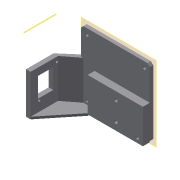
# Autodesk Inventor part: cellSTORM_inverted_Laser_left
Saved by Autodesk Inventor 2019.4 (Build 234330000, 330)
## iProperties
Created: 2020-11-05
Part Number: cellSTORM_inverted_Laser_left
Material: Generic
Document SubType Name: Modeling
Designer: diederichbenedict
Density: 1 g/cm^3
Appearance: Default
Author: diederichbenedict
Autodesk Inventor part; units mm, degrees
ref_plane "Work Plane1" through (0, 0, 0) normal (0, 0, 1) x (1, 0, 0)
sketch "Sketch1" plane through (0, 0, 0) normal (0, 0, 1) x (1, 0, 0)
  circle A0 centre (0, 25) radius 1.95 construction
  circle A1 centre (-25, 0) radius 1.95 construction
  circle A2 centre (-25, -25) radius 1.95 construction
  circle A3 centre (25, 25) radius 1.95 construction
  circle A4 centre (25, -25) radius 1.95 construction
  circle A5 centre (-25, 25) radius 1.95 construction
  circle A6 centre (25, 0) radius 1.95 construction
  circle A7 centre (0, -25) radius 1.95 construction
  line L0 (-28, 30) -> (-30, 28) projected
  line L1 (-30, 28) -> (-30, -28) projected
  line L2 (-30, -28) -> (-28, -30) projected
  line L3 (-28, -30) -> (28, -30) projected
  line L4 (28, -30) -> (30, -28) projected
  line L5 (30, -28) -> (30, 28) projected
  line L6 (30, 28) -> (28, 30) projected
  line L7 (28, 30) -> (-28, 30) projected
  circle A8 centre (25, 25) radius 1.45
  circle A9 centre (25, -25) radius 1.45
  circle A10 centre (-25, -25) radius 1.45
  circle A11 centre (-25, 25) radius 1.45
  circle A12 centre (0, 25) radius 1.95 projected
  circle A13 centre (-25, 0) radius 1.95 projected
  circle A14 centre (-25, -25) radius 1.95 projected
  circle A15 centre (25, 25) radius 1.95 projected
  circle A16 centre (25, -25) radius 1.95 projected
  circle A17 centre (-25, 25) radius 1.95 projected
  circle A18 centre (25, 0) radius 1.95 projected
  circle A19 centre (0, -25) radius 1.95 projected
  line L8 (-28, 30) -> (-30, 28) projected
  line L9 (-30, 28) -> (-30, -28) projected
  line L10 (-30, -28) -> (-28, -30) projected
  line L11 (-28, -30) -> (28, -30) projected
  line L12 (28, -30) -> (30, -28) projected
  line L13 (30, -28) -> (30, 28) projected
  line L14 (30, 28) -> (28, 30) projected
  line L15 (28, 30) -> (-28, 30) projected
  line L16 (-44.5, 28.8555) -> (-44.5, 2)
  line L17 (-44.5, 34) -> (-45.5, 34)
  line L18 (-45.5, 1) -> (-44.5, 1)
  line L19 (-44.5, 34) -> (-30, 34)
  line L20 (-30, 34) -> (-30, 1)
  line L21 (-30, 1) -> (-44.5, 1)
  line L22 (-44.5, 1) -> (-44.5, 34)
  line L23 (-30, 34) -> (-26, 30)
  line L24 (-30, 34) -> (-24.3431, 34) construction
  point P0 (0, 0)
  dimension "d0" = 2.9
  dimension "d1" = 2.9
  dimension "d2" = 2.9
  dimension "d3" = 2.9
  dimension "d6" = 45
  constraints: 18 end point, 4 centre point, 4 horizontal, 3 coincident, 2 parallel, 2 point on line, 1 equal length, 1 perpendicular, 1 vertical, 6 other
  measures "d0" diameter of A8
  measures "d1" diameter of A9
  measures "d2" diameter of A10
  measures "d3" diameter of A11
  measures "d6" angle of L23 L24
ref_plane "Work Plane2" through (-18, -2, 8) normal (0, 0, -1) x (0, 1, 0)
extrude "Extrusion1" add sketch "Sketch1" along normal blind 3 contours L7 L6 L5 L4 L3 L2 L1 L0 | A12 | A13 | A14 | A15 | A16 | A17 | A18 | A19
sketch "Sketch2" plane through (0, 0, 3) normal (0, 0, 1) x (1, 0, 0)
  arc A0 (7.0684, -7) -> (5.4716, -7) centre (6.27, -5.85) ccw
  arc A1 (5.4716, -21) -> (7.0684, -21) centre (6.27, -22.15) ccw
  line L0 (-18.23, -28.95) -> (30, -28.95)
  line L1 (-18.23, 0.95) -> (30, 0.95)
  line L2 (-18.23, 0.95) -> (30, 0.95)
  line L3 (30, 0.95) -> (30, -28.95)
  line L4 (30, -28.95) -> (-18.23, -28.95)
  line L5 (-18.23, -28.95) -> (-18.23, 0.95)
  circle A2 centre (6.27, -5.85) radius 1.4
  circle A3 centre (6.27, -22.15) radius 1.4
  circle A4 centre (25, -25) radius 1.45 projected
  point P0 (0, 0)
  constraints: 12 end point, 4 centre point, 4 point on circle, 3 horizontal, 2 coincident, 2 concentric, 2 parallel, 1 perpendicular, 12 other
ref_plane "Work Plane3" through (-18, -2, 8) normal (0, 0, -1) x (0, 1, 0)
ref_plane "Work Plane6" through (-18.23, -26.95, 9.05) normal (0, 0, -1) x (0, 1, 0)
extrude "Extrusion2" add sketch "Sketch2" along normal up to surface (6.05 mm away)
sketch "Sketch3" plane through (0, 0, 0) normal (0, 0, -1) x (-1, 0, 0)
  line L0 (-30, -28.95) -> (-30, 0.95) projected
  line L1 (18.23, -28.95) -> (-30, -28.95) projected
  line L2 (-30, 0.95) -> (18.23, 0.95) projected
  line L3 (18.23, 0.95) -> (18.23, -28.95) projected
  arc A0 (-5.4716, -7) -> (-7.0684, -7) centre (-6.27, -5.85) ccw
  arc A1 (-7.0684, -21) -> (-5.4716, -21) centre (-6.27, -22.15) ccw
  point P0 (0, 0)
  constraints: 4 point on circle, 2 centre point, 8 other
hole "Hole2" at (6.27, -22.15, 0) at (6.27, -5.85, 0) direction (0, 0, 1) diameter 3.2 depth 20 tip angle 118 counterbore diameter 5 counterbore depth 4
ref_plane "Work Plane4" through (-44.5, 34, 36.7) normal (0, 1, 0) x (0, 0, -1)
sketch "Sketch5" plane through (-44.5, -30, 36.7) normal (0, 1, 0) x (0, 0, -1)
  line L0 (36.7, -72.5) -> (36.7, -16.5) projected
  line L1 (36.7, -16.5) -> (33.7, -16.5) projected
  line L2 (33.7, -72.5) -> (33.7, -16.5) projected
  line L3 (36.7, -72.5) -> (33.7, -72.5) projected
  line L4 (25.7, 0) -> (0, 0) projected
  line L5 (25.7, 0) -> (25.7, 1) projected
  line L6 (0, 1) -> (25.7, 1) projected
  line L7 (0, 0) -> (0, 1) projected
  line L8 (0, 0) -> (24, 0)
  line L9 (24, 0) -> (24, -4)
  line L10 (24, -4) -> (0, -4)
  line L11 (0, -4) -> (0, 0)
  line L12 (24, -4) -> (33.7, -16.5)
  line L13 (36.7, -16.5) -> (36.7, -14.5) projected
  line L14 (36.7, -14.5) -> (36.7, -16.5) projected
  line L15 (24, 0) -> (36.7, -14.5)
  line L16 (36.7, -16.5) -> (33.7, -16.5) projected
  line L17 (36.7, -14.5) -> (36.7, -16.5)
  point P0 (36.7, -44.5)
  dimension "d23" = 24
  dimension "d24" = 4
  constraints: 14 end point, 2 parallel, 2 perpendicular, 1 horizontal
  measures "d23" distance of L9.end L10.end
  measures "d24" distance of L8.end L9.end
ref_plane "Work Plane5" through (-45.5, 1, 28.397) normal (0, -1, 0) x (1, 0, 0)
extrude "Extrusion3" add sketch "Sketch5" along normal up to surface (36 mm away) contours L1 L12 L9 L15 L13 | L10 L11 L4 L9
sketch "Sketch6" plane through (-44.5, -30, 36.7) normal (0, -1, 0) x (-1, 0, 0)
  line L0 (-14.5, 36.7) -> (-72.5, 36.7) projected
  line L1 (-72.5, 36.7) -> (-72.5, 33.7) projected
  line L2 (-16.5, 33.7) -> (-72.5, 33.7) projected
  line L3 (-16.5, 33.7) -> (-4, 24) projected
  line L4 (-4, 24) -> (-4, 0) projected
  line L5 (-4, 0) -> (0, 0) projected
  line L6 (0, 0) -> (0, 24) projected
  line L7 (0, 24) -> (-14.5, 36.7) projected
  line L8 (-26.27, 27.65) -> (-74.5, 27.65) projected
  line L9 (-26.27, 33.7) -> (-26.27, 27.65) projected
  line L10 (-73.55, 33.7) -> (-26.27, 33.7) projected
  line L11 (-73.55, 33.7) -> (-74.5, 33.7) projected
  line L12 (-74.5, 33.7) -> (-74.5, 27.65) projected
  line L13 (-74.5, 27.65) -> (-26.27, 27.65) projected
  line L14 (-4, 0) -> (-26.27, 27.65)
  line L15 (-26.27, 33.7) -> (-26.27, 27.65) projected
  line L16 (-26.27, 27.65) -> (-26.27, 33.7)
  line L17 (-26.27, 33.7) -> (-16.5, 33.7)
  line L18 (-16.5, 33.7) -> (-4, 24)
  line L19 (-4, 24) -> (-4, 0)
  point P0 (-44.5, 36.7)
  constraints: 10 end point, 1 collinear, 1 perpendicular
extrude "Extrusion4" add sketch "Sketch6" against normal blind 2 contours L2 L3 L4 L14 L9
sketch "Sketch7" plane through (-44.5, 6, 36.7) normal (-1, 0, 0) x (0, 0, 1)
  circle A0 centre (-2.7, 2.5) radius 1
  circle A1 centre (-7.7, -25.5) radius 1
  circle A2 centre (-23.2, -4) radius 1
  circle A3 centre (-12.7, -15) radius 2.6486
  line L0 (-6.3458, -6.3489) -> (-19.7341, -6.3489)
  line L1 (-19.7341, -6.3489) -> (-19.7341, -23.6095)
  line L2 (-19.7341, -23.6095) -> (-6.3458, -23.6095)
  line L3 (-6.3458, -23.6095) -> (-6.3458, -6.3489)
  constraints: 8 end point, 4 centre point, 2 parallel, 1 horizontal, 1 perpendicular, 8 other
extrude "Extrusion5" cut sketch "Sketch7" against normal through all contours A0 | A1 | A2 | A3 | L3 L2 L1 L0
sketch "Sketch8" plane through (0, 0, 0) normal (0, 0, -1) x (-1, 0, 0)
  line L0 (-28, 30) -> (28, 30) projected
  line L1 (-30, 28) -> (-28, 30) projected
  line L2 (-30, -28) -> (-30, 28) projected
  line L3 (-28, -30) -> (-30, -28) projected
  line L4 (30, 28) -> (30, 6) projected
  line L5 (30, 6) -> (30, -30) projected
  line L6 (30, -30) -> (-28, -30) projected
  circle A0 centre (25, -25) radius 1.45 projected
  circle A1 centre (-25, 25) radius 1.45 projected
  circle A2 centre (-25, -25) radius 1.45 projected
  circle A3 centre (25, 25) radius 1.45 projected
  line L7 (71, -30) -> (71, -28) projected
  line L8 (71, -30) -> (131, 30)
  line L9 (71, -30) -> (155.8528, -30) construction
  line L10 (-28, 30) -> (28, 30) projected
  line L11 (28, 30) -> (30, 28) projected
  point P0 (0, 0)
  dimension "d31" = 135
  constraints: 4 end point, 2 point on line, 1 equal length, 1 horizontal
  measures "d31" angle of L8 L9
extrude "Extrusion6" [suppressed]
body "Solid1"
